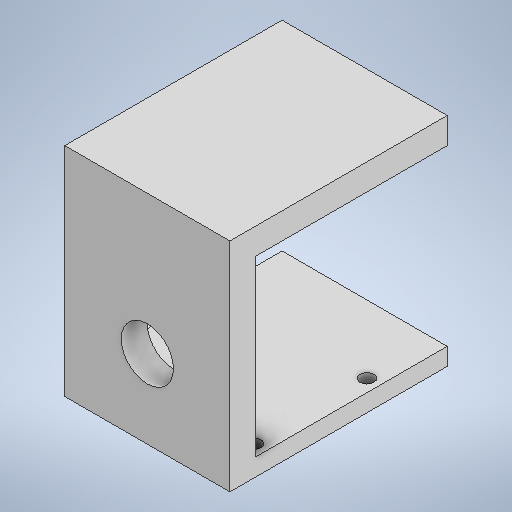
# Autodesk Inventor part: ギアボックス2
Saved by Autodesk Inventor 2026.2 (Build 302298010, 298A)
## iProperties
Created: 2026-05-06
Part Number: ギアボックス2
Material: 一般
Document SubType Name: Modeling
Designer: Yagis
Density: 1 g/cm^3
Appearance: 既定
Author: Yagis
Autodesk Inventor part; units mm, degrees
ref_plane "YZ Plane" through (0, 0, 0) normal (1, 0, 0) x (0, 1, 0)
ref_plane "XZ Plane" through (0, 0, 0) normal (0, 1, 0) x (-1, 0, 0)
ref_plane "XY Plane" through (0, 0, 0) normal (0, 0, 1) x (1, 0, 0)
sketch "スケッチ1" plane through (0, 0, 0) normal (0, 0, 1) x (1, 0, 0)
  line L0 (0, 0) -> (38, 0)
  line L1 (38, 0) -> (38, 24)
  line L2 (38, 24) -> (0, 24)
  line L3 (0, 24) -> (0, 0)
  line L4 (0, 4) -> (38, 4)
  line L5 (13, 33) -> (25, 33)
  line L6 (0, 24) -> (38, 24)
  line L7 (38, 24) -> (38, 44)
  line L8 (38, 44) -> (0, 44)
  line L9 (0, 44) -> (0, 24)
  line L10 (0, 44) -> (38, 44)
  line L11 (38, 44) -> (38, 50)
  line L12 (38, 50) -> (0, 50)
  line L13 (0, 50) -> (0, 44)
  circle A0 centre (19, 33) radius 6
  point P0 (38, 24)
  point P1 (19, 4)
  point P2 (15.6834, 26)
  point P3 (22.3166, 26)
  point P4 (13, 33)
  dimension "d70" = 12
  dimension "d0" = 38
  dimension "d1" = 24
  dimension "d2" = 4
  dimension "d49" = 6
  dimension "d50" = 38
  dimension "d51" = 20
  dimension "d52" = 38
  dimension "d71" = 29
  dimension "d72" = 19
  constraints: 28 end point, 6 parallel, 4 horizontal, 4 perpendicular, 2 midpoint, 2 point on line, 3 other
  measures "d0" distance of L0.start L0.end
  measures "d1" distance of L2.end L0.start
  measures "d2" distance between parallel lines of L0 L4
  measures "d49" distance between parallel lines of L10 L12
  measures "d50" distance between parallel lines of L9 L7
  measures "d51" distance between parallel lines of L8 L2
  measures "d52" distance between parallel lines of L13 L11
  measures "d71" distance of point (19, 4) point (19, 33)
  measures "d72" distance from line of L9 point (19, 33)
extrude "押し出し1" add sketch "スケッチ1" against normal blind 6 contours L3 L4 L1 L0 | L3 L2 L1 L4 | L9 L8 L7 L2 | L13 L12 L11 L8 | A0 L5 | L5 A0
extrude "押し出し2" add sketch "スケッチ1" against normal blind 50 contours L3 L4 L1 L0 | L13 L12 L11 L8
sketch "スケッチ2" plane through (0, 0, 0) normal (0, 0, 1) x (1, 0, 0)
  line L0 (0, 50) -> (0, 0) projected
  line L1 (38, 50) -> (0, 50) projected
  line L2 (38, 0) -> (38, 50) projected
  line L3 (38, 50) -> (0, 50) projected
  line L4 (0, 50) -> (0, 0) projected
  line L5 (0, 0) -> (38, 0) projected
  point P0 (19, 18)
  point P1 (0, 26)
  point P2 (0, 25)
  point P3 (19, 50)
  point P4 (19, 0)
  point P5 (19, 50)
  dimension "d74" = 32
  constraints: 4 midpoint, 2 vertical alignment
  measures "d74" distance from line of point (19, 18) L1
hole "穴1" at (19, 18, 0) direction (0, 0, -1) diameter 12 depth 8.1 tip angle 118
sketch "スケッチ4" plane through (0, 4, -6) normal (0, 1, 0) x (1, 0, 0)
  point P0 (0, -6)
  point P1 (3.1531, 2.3812)
  point P2 (35.1531, 2.3812)
  point P3 (35.1531, 28.3812)
  point P4 (3.1531, 28.3812)
  dimension "d47" = 32
  dimension "d48" = 26
  constraints: 2 horizontal alignment, 2 vertical alignment
  measures "d47" distance of point (35.153, 2.381) point (3.153, 2.381)
  measures "d48" distance of point (35.153, 28.381) point (35.153, 2.381)
hole "穴3" at (3.1531, 4, -8.3812) at (35.1531, 4, -8.3812) at (35.1531, 4, -34.3812) at (3.1531, 4, -34.3812) direction (0, -1, 0) diameter 3.2 depth 8.1 tip angle 118
equation "\"d51\" = d1 - d2"
